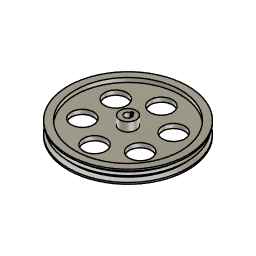
29 (Autodesk Fusion 360 design; units mm, degrees)
Autodesk Fusion 360 part; units mm, degrees
sketch "草图1" plane through (0, 0, 0) normal (1, 0, 0) x (0, 1, 0)
  line L0 (0, 90) -> (0, -60) construction
  line L1 (0, 30) -> (22, 30)
  line L2 (22, 30) -> (22, -30)
  line L3 (22, -30) -> (0, -30)
  line L4 (22, 6) -> (142, 6)
  line L5 (142, 6) -> (142, 17.5)
  line L6 (142, 17.5) -> (161, 17.5)
  line L7 (161, -17.5) -> (142, -17.5)
  line L8 (142, -17.5) -> (142, -6)
  line L9 (142, -6) -> (22, -6)
  line L10 (0, 30) -> (0, -30)
  line L11 (-55, 0) -> (190, 0) construction
  line L12 (161, -17.5) -> (161, -13.4)
  line L13 (161, -13.4) -> (149, -9.2681)
  line L14 (149, -9.2681) -> (149, -2.9268)
  line L15 (149, -2.9268) -> (157.5, 0)
  line L16 (157.5, 0) -> (149, 2.9268)
  line L17 (149, 2.9268) -> (149, 9.2681)
  line L18 (149, 9.2681) -> (161, 13.4)
  line L19 (161, 13.4) -> (161, 17.5)
  line L20 (149, -6.0974) -> (142, -6.0974) construction
  line L21 (149, 6.0974) -> (148, 6.0974)
  line L22 (148, 6.0974) -> (142, 6.0974) construction
  point P0 (149, 6.0974)
  point P1 (149, -6.0974)
  dimension "d1" = 22
  dimension "d2" = 60
  dimension "d3" = 12
  dimension "d5" = 161
  dimension "d6" = 157.5
  dimension "d7" = 149
  dimension "d8" = 13.4
  dimension "d9" = 38
  dimension "d10" = 142
  dimension "d11" = 35
  constraint vertical L0
  constraint coincident L0 L1.start
  constraint perpendicular L0 L1
  constraint perpendicular L1 L2
  constraint coincident L0 L3.end
  constraint perpendicular L0 L3
  constraint coincident L2 L4.start
  constraint perpendicular L2 L4
  constraint perpendicular L4 L5
  constraint perpendicular L5 L6
  constraint perpendicular L7 L8
  constraint coincident L2 L9.end
  constraint perpendicular L2 L9
  constraint horizontal L11
  constraint symmetric L4 L9 L11
  constraint symmetric L1 L3 L11
  constraint symmetric L6 L7 L11
  constraint perpendicular L7 L12
  constraint vertical L14
  constraint coincident L11 L15.end
  constraint perpendicular L11 L17
  constraint symmetric L11 L13 L18
  constraint symmetric L11 L15 L16
  constraint symmetric L11 L14 L17
  constraint perpendicular L11 L19
  constraint symmetric L5 L8 L11
  constraint midpoint L17 P0
  constraint midpoint L14 P1
  constraint coincident P1 L20.start
  constraint coincident L8 L20.end
  constraint perpendicular L8 L20
  constraint coincident P0 L21.start
  constraint perpendicular L17 L21
  constraint coincident L5 L22.end
  constraint perpendicular L5 L22
  constraint symmetric L11 L12.end L18.end
  measures "d1" distance of L1.start L1.end
  measures "d2" distance of L1.end L2.end
  measures "d3" distance of L4 L9
  measures "d5" horizontal distance of L1.start L6.end
  measures "d6" distance of origin L15.end
  measures "d7" horizontal distance of origin L17.end
  measures "d8" vertical distance of L12.end L15.end
  measures "d9" angle of L16 L18
  measures "d10" horizontal distance of origin L5.end
  measures "d11" vertical distance of L6.end L7.start
revolve "旋转1" add sketch "草图1" angle 360 about axis through (0, 0, 90) along (0, 0, -1)
sketch "草图2" plane through (0, 0, 6) normal (0, 0, 1) x (-1, 0, 0)
  circle A0 centre (0, 0) radius 22
  circle A1 centre (0, 0) radius 142
  circle A2 centre (0, -90) radius 30
  circle A3 centre (77.9423, -45) radius 30
  circle A4 centre (77.9423, 45) radius 30
  circle A5 centre (0, 90) radius 30
  circle A6 centre (-77.9423, 45) radius 30
  circle A7 centre (-77.9423, -45) radius 30
  dimension "d13" = 90
  dimension "d14" = 60
  dimension "d16" = 360
  measures "d13" distance of A0.centre A2.centre
  measures "d14" diameter of A2
extrude "拉伸1" cut sketch "草图2" against normal blind 90 contours A2 | A3 | A4 | A5 | A6 | A7
sketch "草图3" plane through (0, 0, 30) normal (0, 0, 1) x (-1, 0, 0)
  circle A0 centre (0, 0) radius 22
  line L0 (3, -9.5394) -> (3, -13.5)
  line L1 (3, -13.5) -> (-3, -13.5)
  line L2 (-3, -13.5) -> (-3, -9.5394)
  line L3 (0, -30) -> (0, 30) construction
  arc A1 (3, -9.5394) -> (-3, -9.5394) centre (0, 0) ccw
  dimension "d19" = 6
  dimension "d20" = 20
  dimension "d21" = 23.5
  constraint concentric A0 A1
  constraint vertical L0
  constraint perpendicular L0 L1
  constraint perpendicular L1 L2
  constraint vertical L3
  constraint symmetric L0 L2 L3
  measures "d19" distance of L0 L2
  measures "d20" diameter of A1
extrude "拉伸2" cut sketch "草图3" against normal blind 110 contours L0 L1 L2 A1
